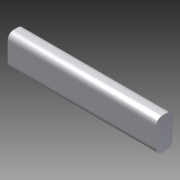
# Autodesk Inventor part: batteri
Saved by Autodesk Inventor 2012 (Build 160160000, 160)
## iProperties
Created: 2012-02-28
Part Number: batteri
Material: Default
Document SubType Name: Modeling
Designer: Grailas
Density: 1 g/cm^3
Author: Grailas
Autodesk Inventor part; units mm, degrees
ref_plane "YZ Plane" through (0, 0, 0) normal (1, 0, 0) x (0, 1, 0)
ref_plane "XZ Plane" through (0, 0, 0) normal (0, 1, 0) x (-1, 0, 0)
ref_plane "XY Plane" through (0, 0, 0) normal (0, 0, 1) x (1, 0, 0)
sketch "Sketch1" plane through (0, 0, 0) normal (0, 0, 1) x (1, 0, 0)
  line L0 (-106, 11.5) -> (106, 11.5)
  line L1 (106, 11.5) -> (106, -11.5)
  line L2 (106, -11.5) -> (-106, -11.5)
  line L3 (-106, -11.5) -> (-106, 11.5)
  point P0 (0, 0)
  point P1 (0, -11.5)
  point P2 (-106, 0)
  dimension "d0" = 212
  dimension "d1" = 23
  constraints: 8 end point, 2 midpoint, 2 parallel, 1 horizontal, 1 horizontal alignment, 1 perpendicular, 1 vertical alignment
  measures "d0" distance of L1.end L2.end
  measures "d1" distance of L0.end L1.end
extrude "Extrusion1" add sketch "Sketch1" along normal blind 46
fillet "Fillet1" radius 10 1 edges at (0, 11.5, 0) curvature continuous yes
fillet "Fillet2" radius 10 3 edges at (0, -11.5, 0) (0, -11.5, 46) (0, 11.5, 46) curvature continuous yes
body "Solid1"
